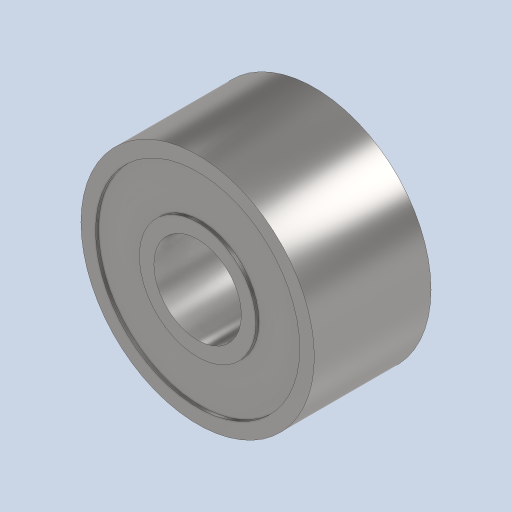
# Autodesk Inventor part: 693ZZ
Saved by Autodesk Inventor 2024 (Build 280153000, 153)
## iProperties
Created: 2023-08-10
Part Number: 693ZZ
Material: ステンレス鋼
Document SubType Name: Modeling
Designer: zegi
Density: 8 g/cm^3
Appearance: 半つや出し
Author: zegi
Autodesk Inventor part; units mm, degrees
ref_plane "YZ Plane" through (0, 0, 0) normal (1, 0, 0) x (0, 1, 0)
ref_plane "XZ Plane" through (0, 0, 0) normal (0, 1, 0) x (-1, 0, 0)
ref_plane "XY Plane" through (0, 0, 0) normal (0, 0, 1) x (1, 0, 0)
sketch "スケッチ1" plane through (0, 0, 0) normal (0, 0, 1) x (1, 0, 0)
  circle A0 centre (0, 0) radius 1.5
  circle A1 centre (0, 0) radius 4
  circle A2 centre (0, 0) radius 2
  circle A3 centre (0, 0) radius 3.5
  dimension "d0" = 3
  dimension "d1" = 8
  dimension "d2" = 4
  dimension "d3" = 0.5
  constraints: 4 centre point, 3 coincident
  measures "d0" diameter of A0
  measures "d1" diameter of A1
  measures "d2" diameter of A2
  measures "d3" radial gap between concentric circles of A1 A3
extrude "押し出し1" add sketch "スケッチ1" along normal blind 2 contours A1 | A2 | A3
extrude "押し出し2" cut sketch "スケッチ1" against normal blind 0.1 from surface at 2 contours A3
mirror "ミラー1" about plane through (0, 0, 0) normal (0, 0, -1) of "押し出し1", "押し出し2"
